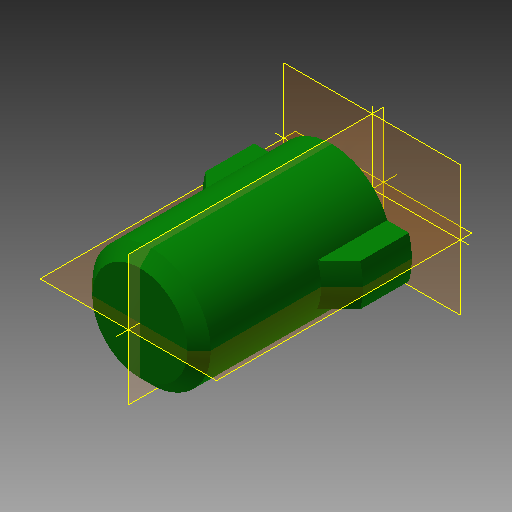
# Autodesk Inventor part: HbThumbLockButton01
Saved by Autodesk Inventor 2018 (Build 220112000, 112)
## iProperties
Created: 2015-09-12
Part Number: HbThumbLockButton01
Material: ABS プラスチック
Document SubType Name: Modeling
Designer: Yamaura
Density: 1.06 g/cm^3
Appearance: 濃い緑
Author: Yamaura
Autodesk Inventor part; units mm, degrees
sketch "スケッチ1" plane through (0, 0, 0) normal (0, 0, 1) x (1, 0, 0)
  circle A0 centre (0, 0) radius 5.1
  dimension "d0" = 10.2
  constraints: 1 centre point, 1 coincident
  measures "d0" diameter of A0
extrude "押し出し1" add sketch "スケッチ1" along normal blind 16.5
sketch "スケッチ3" plane through (0, 0, 0) normal (0, 0, 1) x (1, 0, 0)
  point P0 (0, 0)
sketch "スケッチ4" plane through (0, 0, 0) normal (0, 0, 1) x (1, 0, 0)
  line L0 (-7.0548, -0.8) -> (7.0548, -0.8)
  line L1 (7.0548, 0.8) -> (-7.0548, 0.8)
  line L2 (-8, -1) -> (8, 1) construction
  line L3 (8.9625, -1.2804) -> (-7, 1) construction
  arc A0 (7.0548, -0.8) -> (7.0548, 0.8) centre (0, 0) ccw
  arc A1 (-7.0548, 0.8) -> (-7.0548, -0.8) centre (0, 0) ccw
  dimension "d20" = 0.8
  dimension "d21" = 0.8
  dimension "d25" = 7.1
  dimension "d26" = 7.1
  constraints: 8 end point, 4 point on circle, 2 centre point, 1 coincident, 1 horizontal, 1 midpoint, 1 parallel, 1 point on line
  measures "d20" distance from line of L1 point (0, 0)
  measures "d21" distance from line of L0 point (0, 0)
  measures "d25" radius of A1
  measures "d26" radius of A0
extrude "押し出し3" add sketch "スケッチ4" along normal blind 6
sketch "スケッチ2" plane through (0, 0, 0) normal (0, 0, 1) x (1, 0, 0)
  circle A0 centre (0, 0) radius 3.3
  dimension "d3" = 6.6
  constraints: 1 centre point, 1 coincident
  measures "d3" diameter of A0
extrude "押し出し2" cut sketch "スケッチ2" along normal blind 4.5
sketch "スケッチ5" plane through (0, 0, 4.5) normal (0, 0, -1) x (-1, 0, 0)
  circle A0 centre (0, 0) radius 2
  dimension "d13" = 4
  constraints: 1 centre point, 1 coincident
  measures "d13" diameter of A0
extrude "押し出し4" add sketch "スケッチ5" along normal blind 1.5
chamfer "面取り2" distance 1 angle 45 1 edges at (-5.1, 0, 16.5)
chamfer "面取り3" distance 2 angle 45 1 edges at (-7.1, 0, 6)
chamfer "面取り4" distance 2 angle 45 1 edges at (7.1, 0, 6)
move faces "移動1" translate (0, 1, 0) faces at (6.3821, 0.8, 1.3334) (-6.3821, 0.8, 1.3334)
move faces "移動2" translate (0, -1, 0) faces at (-6.3821, -0.8, 1.3334) (6.3821, -0.8, 1.3334)
offset faces "サイズ1" outward -0.2 faces at (7.086, 0.4451, 2.6667) (-7.086, -0.4451, 2.6667)
scale "尺度2" factors (0.69, 0.69, 0.69) then translate (0, 0, 2.4025) bodies 1
offset faces "サイズ3" outward -0.2 faces at (2.2475, -0.3653, 4.4725)
